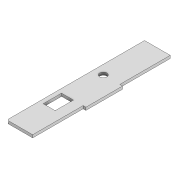
# Autodesk Inventor part: Lateral BNC
Saved by Autodesk Inventor 2020 (Build 240168000, 168)
## iProperties
Created: 2020-11-07
Part Number: Lateral BNC
Material: Generic
Document SubType Name: Modeling
Designer: ferrerx
Density: 1 g/cm^3
Appearance: Default
Author: ferrerx
Autodesk Inventor part; units mm, degrees
ref_plane "YZ Plane" through (0, 0, 0) normal (1, 0, 0) x (0, 1, 0)
ref_plane "XZ Plane" through (0, 0, 0) normal (0, 1, 0) x (-1, 0, 0)
ref_plane "XY Plane" through (0, 0, 0) normal (0, 0, 1) x (1, 0, 0)
sketch "Sketch1" plane through (0, 0, 0) normal (0, 1, 0) x (-1, 0, 0)
  line L0 (0, 0) -> (28, 0)
  line L1 (28, 0) -> (28, -150)
  line L2 (28, -150) -> (0, -150)
  line L3 (0, -150) -> (0, 0)
  line L4 (0, -55) -> (-3, -55)
  line L5 (-3, -55) -> (-3, -95)
  line L6 (-3, -95) -> (0, -95)
  line L7 (0, -95) -> (0, -55)
  line L8 (28, -75) -> (0, -75) construction
  line L9 (-3, -75) -> (0, -75) construction
  point P0 (0, -95)
  dimension "d0" = 150
  dimension "d1" = 3
  dimension "d2" = 40
  dimension "d3" = 28
  constraints: 20 end point, 4 midpoint, 4 parallel, 2 horizontal, 2 perpendicular, 1 collinear, 1 point on line
  measures "d0" distance of L2.end L0.start
  measures "d1" distance of L5.end L6.end
  measures "d2" distance of L4.end L5.end
  measures "d3" distance of L1.end L2.end
extrude "Extrusion1" add sketch "Sketch1" along normal blind 3
sketch "Sketch3" plane through (0, 3, 0) normal (0, 1, 0) x (1, 0, 0)
  circle A0 centre (-18, 95) radius 3.9
  line L0 (-28, 150) -> (-28, 0) projected
  line L1 (0, 95) -> (0, 150) projected
  line L2 (-28, 0) -> (0, 0) projected
  line L3 (0, 150) -> (-28, 150) projected
  dimension "d18" = 7.8
  dimension "d20" = 18
  dimension "d24" = 55
  constraints: 1 centre point
  measures "d18" diameter of A0
  measures "d20" distance from line of L1 A0.centre
  measures "d24" distance from line of L3 A0.centre
extrude "Extrusion3" cut sketch "Sketch3" against normal blind 3
sketch "Sketch4" plane through (0, 0, 0) normal (0, -1, 0) x (1, 0, 0)
  line L0 (-10.5, -55) -> (-23.5, -55)
  line L1 (-23.5, -55) -> (-23.5, -35)
  line L2 (-23.5, -35) -> (-10.5, -35)
  line L3 (-10.5, -35) -> (-10.5, -55)
  line L4 (-10.5, -55) -> (-23.5, -35) construction
  line L5 (-23.5, -55) -> (-10.5, -35) construction
  line L6 (-28, 0) -> (0, 0) projected
  point P0 (-17, -45)
  dimension "d25" = 20
  dimension "d26" = 13
  dimension "d27" = 45
  constraints: 12 end point, 2 midpoint, 2 parallel, 1 horizontal, 1 perpendicular
  measures "d25" distance of L2.end L0.start
  measures "d26" distance of L1.end L2.end
  measures "d27" distance from line of L6 point (-17, -45)
extrude "Extrusion4" cut sketch "Sketch4" against normal blind 10
fillet "Fillet1" radius 2 1 edges at (-28, 1.5, 0)
body "Solid1"
